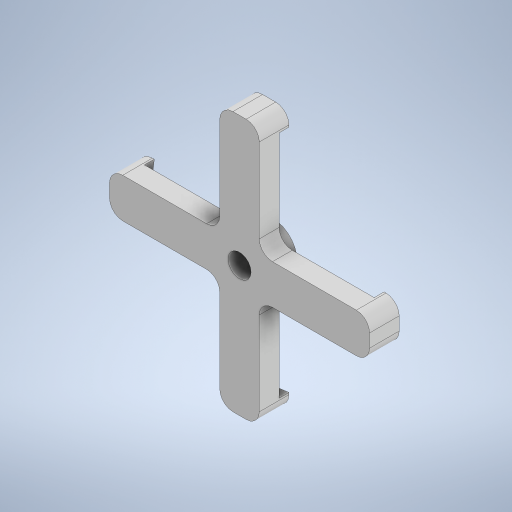
# Autodesk Inventor part: gora
Saved by Autodesk Inventor 2023 (Build 270158000, 158)
## iProperties
Created: 2023-08-20
Part Number: gora
Material: Ogólny
Document SubType Name: Modeling
Designer: Kamil
Density: 1 g/cm^3
Appearance: Domyślna
Author: Kamil
Autodesk Inventor part; units mm, degrees
ref_plane "YZ Plane" through (0, 0, 0) normal (1, 0, 0) x (0, 1, 0)
ref_plane "XZ Plane" through (0, 0, 0) normal (0, 1, 0) x (-1, 0, 0)
ref_plane "XY Plane" through (0, 0, 0) normal (0, 0, 1) x (1, 0, 0)
sketch "Szkic1" plane through (0, 0, 0) normal (0, 0, 1) x (1, 0, 0)
  circle A0 centre (0, 0) radius 17.5 projected
  circle A1 centre (0, 0) radius 15 projected
  line L0 (-3, -17.2409) -> (3, -17.2409)
  line L1 (3, -17.2409) -> (3, 17.2409)
  line L2 (3, 17.2409) -> (-3, 17.2409)
  line L3 (-3, 17.2409) -> (-3, -17.2409)
  line L4 (-3, -17.2409) -> (3, 17.2409) construction
  line L5 (3, -17.2409) -> (-3, 17.2409) construction
  line L6 (17.2409, 3) -> (-17.2409, 3)
  line L7 (-17.2409, 3) -> (-17.2409, -3)
  line L8 (-17.2409, -3) -> (17.2409, -3)
  line L9 (17.2409, -3) -> (17.2409, 3)
  line L10 (17.2409, 3) -> (-17.2409, -3) construction
  line L11 (-17.2409, 3) -> (17.2409, -3) construction
  circle A2 centre (0, 0) radius 1.75
  point P0 (-3, 3)
  point P1 (-3, -3)
  point P2 (3, -3)
  point P3 (3, 3)
  dimension "d0" = 6
  dimension "d1" = 6
  dimension "d2" = 3.5
  constraints: 24 end point, 4 midpoint, 4 parallel, 2 horizontal, 2 perpendicular, 2 point on circle, 1 centre point, 1 coincident
  measures "d0" distance of L2.end L1.end
  measures "d1" distance of L7.end L6.end
  measures "d2" diameter of A2
extrude "Wyciągnięcie proste1" add sketch "Szkic1" along normal blind 3 contours L9 L8 A1 L6 | L1 A1 L3 L2 | A1 L8 L1 L6 | L0 L3 A1 L1 | L1 L6 L3 A1 | L1 L8 L3 L6 | A1 L3 L8 L1 | L6 A1 L8 L7 | L3 L8 A1 L6 | A2
sketch "Szkic2" plane through (0, 0, 3) normal (0, 0, 1) x (1, 0, 0)
  circle A0 centre (0, 0) radius 1.75
  dimension "d5" = 3.5
  constraints: 1 centre point, 1 coincident
  measures "d5" diameter of A0
extrude "Wyciągnięcie proste2" cut sketch "Szkic2" against normal through all
sketch "Szkic3" plane through (0, 0, 0) normal (0, 0, -1) x (-1, 0, 0)
  circle A0 centre (0, 0) radius 1.75
  circle A1 centre (0, 0) radius 3.75
  dimension "d8" = 2
  constraints: 2 centre point, 1 coincident
  measures "d8" radial gap between concentric circles of A0 A1
ref_plane "Płaszczyzna konstrukcyjna1" through (-11.5, -11.5, -2) normal (0, 0, -1) x (0, 1, 0)
extrude "Wyciągnięcie proste3" add sketch "Szkic3" along normal up to surface (2 mm away)
sketch "Szkic4" plane through (0, 0, 3) normal (0, 0, 1) x (1, 0, 0)
  circle A0 centre (0, 0) radius 17.5 projected
  circle A1 centre (0, 0) radius 1.75 projected
  line L0 (-17.2409, 3) -> (-17.2409, -3) projected
  line L1 (-17.2409, -3) -> (-3, -3) projected
  line L2 (-3, -3) -> (-3, -17.2409) projected
  line L3 (-3, -17.2409) -> (3, -17.2409) projected
  line L4 (3, -17.2409) -> (3, -3) projected
  line L5 (3, -3) -> (17.2409, -3) projected
  line L6 (17.2409, -3) -> (17.2409, 3) projected
  line L7 (17.2409, 3) -> (3, 3) projected
  line L8 (3, 3) -> (3, 17.2409) projected
  line L9 (3, 17.2409) -> (-3, 17.2409) projected
  line L10 (-3, 17.2409) -> (-3, 3) projected
  line L11 (-3, 3) -> (-17.2409, 3) projected
  line L12 (17.2409, 3) -> (3, 3) projected
  line L13 (17.2409, 3) -> (19.7409, 3)
  line L14 (19.7409, 3) -> (19.7409, -3)
  line L15 (19.7409, -3) -> (17.2409, -3)
  line L16 (17.2409, -3) -> (17.2409, 3)
  line L17 (-3, 3) -> (-17.2409, 3) projected
  line L18 (-17.2409, 3) -> (-19.7409, 3)
  line L19 (-19.7409, 3) -> (-19.7409, -3)
  line L20 (-19.7409, -3) -> (-17.2409, -3)
  line L21 (-17.2409, -3) -> (-17.2409, 3)
  line L22 (-3, -17.2409) -> (3, -17.2409)
  line L23 (3, -17.2409) -> (3, -19.7409)
  line L24 (3, -19.7409) -> (-3, -19.7409)
  line L25 (-3, -19.7409) -> (-3, -17.2409)
  line L26 (3, 17.2409) -> (-3, 17.2409)
  line L27 (-3, 17.2409) -> (-3, 19.7409)
  line L28 (-3, 19.7409) -> (3, 19.7409)
  line L29 (3, 19.7409) -> (3, 17.2409)
  dimension "d11" = 2.5
  dimension "d12" = 2.5
  dimension "d13" = 2.5
  dimension "d14" = 2.5
  constraints: 32 end point, 8 parallel, 4 horizontal, 4 perpendicular, 1 point on line
  measures "d11" distance of L14.end L15.end
  measures "d12" distance of L20.end L19.end
  measures "d13" distance of L22.end L23.end
  measures "d14" distance of L26.end L27.end
extrude "Wyciągnięcie proste4" add sketch "Szkic4" against normal blind 3 contours A0 L6 | A0 L13 L14 L15 | L9 A0 | A0 L27 L28 L29 | L23 L24 L25 A0 | A0 L3 | L0 A0 | A0 L20 L19 L18
sketch "Szkic5" plane through (0, 0, 0) normal (0, 0, -1) x (-1, 0, 0)
  circle A0 centre (0, 0) radius 17.5 projected
  circle A1 centre (0, 0) radius 3.75 projected
  line L0 (3, 3) -> (19.7409, 3) projected
  line L1 (3, 3) -> (3, 19.7409) projected
  line L2 (3, 19.7409) -> (-3, 19.7409) projected
  line L3 (-3, 3) -> (-3, 19.7409) projected
  line L4 (-3, 3) -> (-19.7409, 3) projected
  line L5 (-19.7409, 3) -> (-19.7409, -3) projected
  line L6 (-3, -3) -> (-19.7409, -3) projected
  line L7 (-3, -3) -> (-3, -19.7409) projected
  line L8 (-3, -19.7409) -> (3, -19.7409) projected
  line L9 (3, -3) -> (3, -19.7409) projected
  line L10 (3, -3) -> (19.7409, -3) projected
  line L11 (19.7409, -3) -> (19.7409, 3) projected
  circle A2 centre (0, 0) radius 17.7
  point P0 (3, -17.4439)
  point P1 (-3, -17.4439)
  point P2 (17.4439, 3)
  point P3 (17.4439, -3)
  point P4 (-17.4439, -3)
  point P5 (-17.4439, 3)
  point P6 (-3, 17.4439)
  point P7 (3, 17.4439)
  dimension "d17" = 0.2
  constraints: 1 centre point
  measures "d17" radial gap between concentric circles of A0 A2
extrude "Wyciągnięcie proste5" add sketch "Szkic5" along normal blind 1.5 contours L0 L11 L10 A2 | A2 L3 L2 L1 | L9 L8 L7 A2 | A2 L6 L5 L4
fillet "Zaokrąglenie1" radius 2 19 edges at (-3, -3, 1.5) (-3, -19.7409, 1.5) (-3, -19.7409, -0.75) (-19.7409, -3, 1.5) (-19.7409, -3, -0.75) (3, -19.7409, 1.5) (3, -19.7409, -0.75) (3, -3, 1.5) (19.7409, -3, 1.5) (19.7409, -3, -0.75) (19.7409, 3, 1.5) (19.7409, 3, -0.75) (3, 3, 1.5) (3, 19.7409, 1.5) (3, 19.7409, -0.75) (-3, 19.7409, 1.5) (-3, 19.7409, -0.75) (-19.7409, 3, 1.5) (-19.7409, 3, -0.75)
fillet "Zaokrąglenie2" radius 2 1 edges at (-3, 3, 1.5)
